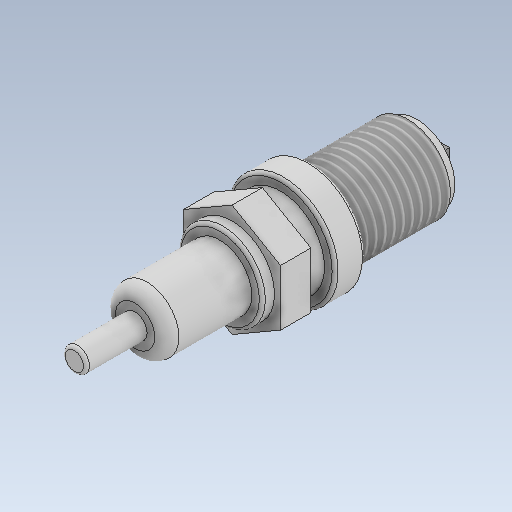
# Autodesk Inventor part: Peça24
Saved by Autodesk Inventor 2021 (Build 250183000, 183)
## iProperties
Category: 41
Created: 2021-07-19
Part Number: Peça24
Material: Genérico
Document SubType Name: Modeling
Designer: Giovanni
Density: 1 g/cm^3
Appearance: Padrão
User Status: 1:1
Author: Giovanni
Keywords: 19
Autodesk Inventor part; units mm, degrees
ref_plane "YZ Plane" through (0, 0, 0) normal (1, 0, 0) x (0, 1, 0)
ref_plane "XZ Plane" through (0, 0, 0) normal (0, 1, 0) x (-1, 0, 0)
ref_plane "XY Plane" through (0, 0, 0) normal (0, 0, 1) x (1, 0, 0)
sketch "Esboço1" plane through (0, 0, 0) normal (0, 0, 1) x (1, 0, 0)
  line L0 (0, 9.2376) -> (8, 4.6188)
  line L1 (8, 4.6188) -> (8, -4.6188)
  line L2 (8, -4.6188) -> (0, -9.2376)
  line L3 (0, -9.2376) -> (-8, -4.6188)
  line L4 (-8, -4.6188) -> (-8, 4.6188)
  line L5 (-8, 4.6188) -> (0, 9.2376)
  point P0 (0, 0)
  point P1 (0, 0)
  dimension "d0" = 16
  constraints: 12 end point, 1 coincident, 13 other
  measures "d0" distance between parallel lines of L1 L4
extrude "Extrusão1" add sketch "Esboço1" along normal blind 5
sketch "Esboço2" plane through (0, 0, 0) normal (0, 0, -1) x (-1, 0, 0)
  circle A0 centre (0, 0) radius 7.25
  dimension "d3" = 14.5
  constraints: 1 centre point, 1 coincident
  measures "d3" diameter of A0
extrude "Extrusão2" add sketch "Esboço2" along normal blind 3
sketch "Esboço3" plane through (0, 0, -3) normal (0, 0, -1) x (-1, 0, 0)
  circle A0 centre (0, 0) radius 9
  dimension "d6" = 18
  constraints: 1 centre point, 1 coincident
  measures "d6" diameter of A0
extrude "Extrusão3" add sketch "Esboço3" along normal blind 5
sketch "Esboço4" plane through (0, 0, -8) normal (0, 0, -1) x (-1, 0, 0)
  circle A0 centre (0, 0) radius 6
  dimension "d9" = 12
  constraints: 1 centre point, 1 coincident
  measures "d9" diameter of A0
extrude "Extrusão4" add sketch "Esboço4" along normal blind 1
sketch "Esboço5" plane through (0, 0, -9) normal (0, 0, -1) x (-1, 0, 0)
  circle A0 centre (0, 0) radius 7
  dimension "d12" = 14
  constraints: 1 centre point, 1 coincident
  measures "d12" diameter of A0
extrude "Extrusão5" add sketch "Esboço5" along normal blind 15
sketch "Esboço6" plane through (0, 0, -24) normal (0, 0, -1) x (-1, 0, 0)
  circle A0 centre (0, 0) radius 6.25
  dimension "d15" = 12.5
  constraints: 1 centre point, 1 coincident
  measures "d15" diameter of A0
extrude "Extrusão6" add sketch "Esboço6" along normal blind 1.5
sketch "Esboço7" plane through (0, 0, -25.5) normal (0, 0, -1) x (-1, 0, 0)
  circle A0 centre (0, 0) radius 4.75
  dimension "d18" = 9.5
  constraints: 1 centre point, 1 coincident
  measures "d18" diameter of A0
extrude "Extrusão7" cut sketch "Esboço7" against normal blind 11.5
sketch "Esboço8" plane through (0, 0, -14) normal (0, 0, -1) x (-1, 0, 0)
  circle A0 centre (0, 0) radius 2
  dimension "d21" = 4
  constraints: 1 centre point, 1 coincident
  measures "d21" diameter of A0
extrude "Extrusão8" add sketch "Esboço8" along normal blind 13
sketch "Esboço9" plane through (0, 0, 0) normal (0, 1, 0) x (-1, 0, 0)
  line L0 (4.75, -25.5) -> (4.75, -14) projected
  line L1 (4.75, -25.5) -> (4.75, -26.5)
  line L2 (-6.25, -25.5) -> (6.25, -25.5) projected
  line L3 (5.95, -25.5) -> (5.95, -26.5)
  line L4 (3.55, -27.7) -> (-2, -27.7)
  line L5 (-2, -27.7) -> (-2, -28.9)
  line L6 (-2, -28.9) -> (3.55, -28.9)
  arc A0 (3.55, -27.7) -> (4.75, -26.5) centre (3.55, -26.5) ccw
  arc A1 (3.55, -28.9) -> (5.95, -26.5) centre (3.55, -26.5) ccw
  line L7 (-2, -27) -> (2, -27) projected
  line L8 (5.95, -25.5) -> (4.75, -25.5)
  point P0 (0, 0)
  dimension "d24" = 1.2
  dimension "d25" = 2.4
  dimension "d26" = 0.7
  dimension "d27" = 1.2
  dimension "d28" = 1.2
  dimension "d29" = 2
  constraints: 12 end point, 4 point on circle, 4 tangent, 2 centre point, 2 horizontal, 2 perpendicular, 2 point on line, 2 vertical
  measures "d24" radius of A0
  measures "d25" radius of A1
  measures "d26" distance between parallel lines of L4 L7
  measures "d27" distance of L4.end L5.end
  measures "d28" distance between parallel lines of L1 L3
  measures "d29" distance from line of point (0, 0) L5
extrude "Extrusão9" add sketch "Esboço9" along normal mid plane 3
sketch "Esboço10" plane through (0, 0, 5) normal (0, 0, 1) x (1, 0, 0)
  circle A0 centre (0, 0) radius 7
  dimension "d32" = 14
  constraints: 1 centre point, 1 coincident
  measures "d32" diameter of A0
extrude "Extrusão10" add sketch "Esboço10" along normal blind 2
sketch "Esboço11" plane through (0, 0, 7) normal (0, 0, 1) x (1, 0, 0)
  circle A0 centre (0, 0) radius 5.25
  dimension "d35" = 10.5
  constraints: 1 centre point, 1 coincident
  measures "d35" diameter of A0
extrude "Extrusão11" add sketch "Esboço11" along normal blind 14
sketch "Esboço12" plane through (0, 0, 21) normal (0, 0, 1) x (1, 0, 0)
  circle A0 centre (0, 0) radius 2
  dimension "d38" = 4
  constraints: 1 centre point, 1 coincident
  measures "d38" diameter of A0
extrude "Extrusão12" add sketch "Esboço12" along normal blind 10
fillet "Arredondamento1" radius 0.5 4 edges at (-2, 0, 31) (-7, 0, 7) (9, 0, -3) (9, 0, -8)
fillet "Arredondamento2" radius 2 1 edges at (-5.25, 0, 21)
thread "Rosca1" size "M14x1.5" class "6g" standard "ANSI Metric M Profile" full length
